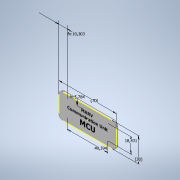
# Autodesk Inventor part: Marking
Saved by Autodesk Inventor 2022 (Build 260153000, 153)
## iProperties
Created: 2021-12-10
Part Number: Marking
Material: Generic
Document SubType Name: Modeling
Designer: Viktor
Density: 1 g/cm^3
Appearance: Default
Author: Viktor
Autodesk Inventor part; units mm, degrees
ref_plane "YZ Plane" through (0, 0, 0) normal (1, 0, 0) x (0, 1, 0)
ref_plane "XZ Plane" through (0, 0, 0) normal (0, 1, 0) x (-1, 0, 0)
ref_plane "XY Plane" through (0, 0, 0) normal (0, 0, 1) x (1, 0, 0)
sketch "Sketch1" plane through (0, 0, 0) normal (0, 0, 1) x (1, 0, 0)
  line L0 (-35, -15) -> (35, -15)
  line L1 (35, -15) -> (35, 15)
  line L2 (35, 15) -> (-35, 15)
  line L3 (-35, 15) -> (-35, -15)
  line L4 (-35, -15) -> (35, 15) construction
  line L5 (35, -15) -> (-35, 15) construction
  point P0 (0, 0)
  dimension "d0" = 70
  dimension "d1" = 30
  constraints: 12 end point, 2 midpoint, 2 parallel, 1 horizontal, 1 perpendicular
  measures "d0" distance of L1.end L2.end
  measures "d1" distance between parallel lines of L0 L2
extrude "Extrusion1" add sketch "Sketch1" along normal blind 2
fillet "Fillet1" radius 5 4 edges at (35, 15, 1) (-35, 15, 1) (35, -15, 1) (-35, -15, 1)
sketch "Sketch2" plane through (0, 0, 2) normal (0, 0, 1) x (1, 0, 0)
  line L0 (-24.6971, 9.2157) -> (24.6971, 9.2157) construction
  line L1 (24.6971, 9.2157) -> (24.6971, -9.2157) construction
  line L2 (24.6971, -9.2157) -> (-24.6971, -9.2157) construction
  line L3 (-24.6971, -9.2157) -> (-24.6971, 9.2157) construction
  line L4 (30, 15) -> (-30, 15) projected
  line L5 (-30, -15) -> (30, -15) projected
  line L6 (-35, 10) -> (-35, -10) projected
  line L7 (35, -10) -> (35, 10) projected
  point P0 (0, 0)
  dimension "d5" = 5.7843
  dimension "d6" = 18.4313
  dimension "d7" = 30
  dimension "d8" = 10.3029
  dimension "d9" = 70
  dimension "d10" = 49.3942
  constraints: 2 other
  measures "d5" distance between parallel lines of L4 L0
  measures "d6" distance between parallel lines of L0 L2
  measures "d7" distance between parallel lines of L5 L4
  measures "d8" distance between parallel lines of L6 L3
  measures "d9" distance between parallel lines of L7 L6
  measures "d10" distance between parallel lines of L1 L3
equation "\"d5\" = -0.5 * d6 + 0.5 * d7"
equation "\"d8\" = -0.5 * d10 + 0.5 * d9"
body "Solid1"
